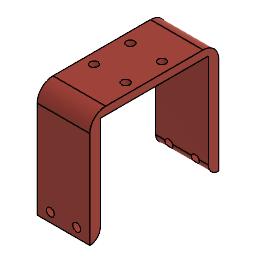
Soporte Inferior (Autodesk Fusion 360 design; units mm, degrees)
Autodesk Fusion 360 part; units mm, degrees
note: some values were not read from the file. Set by a fixed rule: which face or edge a step refers to.
sketch "Boceto1" plane through (0, 0, 0) normal (0, 0, 1) x (1, 0, 0)
  line L0 (0, 0) -> (20, 0)
  line L1 (20, 0) -> (20, 21.8)
  line L2 (20, 21.8) -> (0, 21.8)
  line L3 (0, 21.8) -> (0, 0)
  line L4 (0, 21.8) -> (4, 21.8)
  line L5 (4, 21.8) -> (4, 17.8)
  line L6 (0, 0) -> (4, 0)
  line L7 (4, 0) -> (4, 4)
  circle A0 centre (4, 17.8) radius 1.5
  circle A1 centre (4, 4) radius 1.5
  line L8 (20, 21.8) -> (20, 17.8)
  line L9 (20, 17.8) -> (16, 17.8)
  line L10 (20, 0) -> (16, 0)
  line L11 (16, 0) -> (16, 4)
  circle A2 centre (16, 17.8) radius 1.5
  circle A3 centre (16, 4) radius 1.5
  dimension "d1" = 20
  dimension "d2" = 21.8
  dimension "d3" = 4
  dimension "d4" = 4
  dimension "d5" = 4
  dimension "d6" = 4
  dimension "d7" = 3
  dimension "d8" = 3
  dimension "d36" = 4
  dimension "d37" = 4
  dimension "d38" = 4
  dimension "d39" = 4
  dimension "d40" = 3
  dimension "d41" = 3
  constraint horizontal L0
  constraint vertical L1
  constraint horizontal L2
  constraint vertical L3
  constraint coincident L0.start L3.end
  constraint perpendicular L3 L4
  constraint perpendicular L2 L5
  constraint perpendicular L3 L6
  constraint perpendicular L0 L7
  constraint coincident L5.end A0.centre
  constraint coincident L7.end A1.centre
  constraint perpendicular L2 L8
  constraint perpendicular L8 L9
  constraint perpendicular L1 L10
  constraint perpendicular L0 L11
  constraint coincident L9.end A2.centre
  constraint coincident L11.end A3.centre
  measures "d1" distance of L0.start L0.end
  measures "d2" distance of L0.start L2.end
  measures "d3" distance of L2.end L4.end
  measures "d4" distance of L4.end L5.end
  measures "d5" distance of L0.start L6.end
  measures "d6" distance of L6.end L7.end
  measures "d7" diameter of A0
  measures "d8" diameter of A1
  measures "d36" distance of L1.end L8.end
  measures "d37" distance of L8.end L9.end
  measures "d38" distance of L0.end L10.end
  measures "d39" distance of L10.end L11.end
  measures "d40" diameter of A2
  measures "d41" diameter of A3
extrude "Extruir1" add sketch "Boceto1" against normal blind 3 makes body 1
move_face "CarasDesfase1" offset 13.6 2 faces at (17.3333, 0, -1) (2.6667, 21.8, -1) on bodies 1
sketch "Boceto4" plane through (0, 0, -3) normal (0, 0, -1) x (1, 0, 0)
  circle A0 centre (16, -17.8) radius 1.5
  circle A1 centre (16, -4) radius 1.5
  circle A2 centre (4, -17.8) radius 1.5
  circle A3 centre (4, -4) radius 1.5
  line L0 (0, -35.4) -> (20, -35.4)
  line L1 (20, -35.4) -> (20, 13.6)
  line L2 (20, 13.6) -> (0, 13.6)
  line L3 (0, 13.6) -> (0, -35.4)
  line L4 (20, 13.6) -> (0, 13.6)
  line L5 (0, 13.6) -> (0, 9.6)
  line L6 (0, 9.6) -> (20, 9.6)
  line L7 (20, 9.6) -> (20, 13.6)
  line L8 (20, -35.4) -> (0, -35.4)
  line L9 (0, -35.4) -> (0, -31.4)
  line L10 (0, -31.4) -> (20, -31.4)
  line L11 (20, -31.4) -> (20, -35.4)
  dimension "d43" = 4
  dimension "d44" = 4
  constraint horizontal L4
  constraint vertical L5
  constraint horizontal L6
  constraint vertical L7
  constraint coincident L1.end L2.start
  constraint horizontal L8
  constraint vertical L9
  constraint horizontal L10
  constraint vertical L11
  constraint coincident L0.end L1.start
  measures "d43" distance of L1.end L6.end
  measures "d44" distance of L0.end L10.end
extrude "Extruir4" add sketch "Boceto4" along normal blind 37.85 contours L0 L1 L3 L8 L9 L10 L11 | L1 L2 L3 L4 L5 L6 L7 bodies 1
sketch "Boceto5" plane through (0, -13.6, 0) normal (0, -1, 0) x (1, 0, 0)
  line L0 (20, 0) -> (0, 0)
  line L1 (0, 0) -> (0, -40.85)
  line L2 (0, -40.85) -> (20, -40.85)
  line L3 (20, -40.85) -> (20, 0)
  line L4 (20, -40.85) -> (-0.0041, -40.85)
  line L5 (-0.0041, -40.85) -> (-0.0041, -37.85)
  line L6 (-0.0041, -37.85) -> (20, -37.85)
  line L7 (20, -37.85) -> (20, -40.85)
  dimension "d47" = 3
  constraint horizontal L4
  constraint vertical L5
  constraint horizontal L6
  constraint vertical L7
  constraint coincident L2.end L3.start
  measures "d47" distance of L2.end L6.end
sketch "Boceto6" plane through (0, 35.4, 0) normal (0, 1, 0) x (-1, 0, 0)
  line L0 (0, 0) -> (-20, 0)
  line L1 (-20, 0) -> (-20, -40.85)
  line L2 (-20, -40.85) -> (0, -40.85)
  line L3 (0, -40.85) -> (0, 0)
  line L4 (-20, -40.85) -> (0.0041, -40.85)
  line L5 (0.0041, -40.85) -> (0.0041, -37.85)
  line L6 (0.0041, -37.85) -> (-20, -37.85)
  line L7 (-20, -37.85) -> (-20, -40.85)
  dimension "d48" = 3
  constraint horizontal L4
  constraint vertical L5
  constraint horizontal L6
  constraint vertical L7
  constraint coincident L1.end L2.start
  measures "d48" distance of L1.end L6.end
sketch "Boceto7" plane through (0, -13.6, 0) normal (0, -1, 0) x (1, 0, 0)
  line L0 (20, 0) -> (0, 0)
  line L1 (0, 0) -> (0, -40.85)
  line L2 (0, -40.85) -> (20, -40.85)
  line L3 (20, -40.85) -> (20, 0)
  line L4 (5, -40.85) -> (5, -39.35)
  line L5 (20, -40.85) -> (15, -40.85)
  line L6 (15, -40.85) -> (15, -39.35)
  circle A0 centre (5, -39.35) radius 1.5
  circle A1 centre (15, -39.35) radius 1.5
  line L7 (0, -40.85) -> (5, -40.85)
  dimension "d54" = 1.5
  dimension "d55" = 5
  dimension "d56" = 1.5
  dimension "d57" = 3
  dimension "d58" = 3
  dimension "d67" = 5
  constraint coincident L2 L4.start
  constraint perpendicular L2 L4
  constraint coincident L2.end L3.start
  constraint perpendicular L3 L5
  constraint perpendicular L5 L6
  constraint coincident L4.end A0.centre
  constraint coincident L6.end A1.centre
  constraint coincident L1.end L2.start
  constraint perpendicular L1 L7
  constraint coincident L4.start L7.end
  measures "d54" distance of L4.start L4.end
  measures "d55" distance of L2.end L5.end
  measures "d56" distance of L5.end L6.end
  measures "d57" diameter of A0
  measures "d58" diameter of A1
  measures "d67" distance of L1.end L4.start
extrude "Extruir8" add 2 faces at (13.3333, -10.9333, -40.85) (6.6667, 32.7333, -40.85) along direction (0, 0, -1) blind 2 on bodies 1 bodies 1
extrude "Extruir7" cut sketch "Boceto7" against normal up to surface (49 mm away) contours A0 | A1 bodies 1
fillet "Empalme3" radius 6 2 edges at (10, -13.6, 0) (10, 35.4, 0) on bodies 1
fillet "Empalme4" radius 4 2 edges at (10, -9.6, -42.85) (10, 31.4, -42.85) on bodies 1
copy_body "Cuerpo - > Comp.2" bodies 1 removing the originals makes body 2 in component "Soporte inferior"
component "Soporte inferior" placed x (1, 0, 0) y (0, 1, 0) z (0, 0, 1) at (0, 0, 0)
named bodies: "Soporte inferior"
